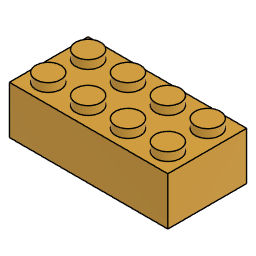
LEGO (Autodesk Fusion 360 design; units mm, degrees)
Autodesk Fusion 360 part; units mm, degrees
sketch "Sketch1" plane through (0, 0, 0) normal (0, 0, 1) x (1, 0, 0) in component "LEGO"
  line L0 (0, 0) -> (31.8, 0)
  line L1 (31.8, 0) -> (31.8, 15.8)
  line L2 (31.8, 15.8) -> (0, 15.8)
  line L3 (0, 15.8) -> (0, 0)
  dimension "d1" = 31.8
  dimension "d2" = 15.8
  constraint horizontal L0
  constraint vertical L1
  constraint horizontal L2
  constraint vertical L3
  constraint coincident L0.start L3.end
  measures "d1" distance of L0.start L0.end
  measures "d2" distance of L0.start L2.end
extrude "Extrude1" add sketch "Sketch1" along normal blind 9.6 makes body 1 in component "LEGO"
sketch "Sketch2" plane through (0, 0, 9.6) normal (0, 0, 1) x (-1, 0, 0) in component "LEGO"
  line L0 (0, -15.8) -> (0, 0)
  line L1 (0, 0) -> (-31.8, 0)
  line L2 (-31.8, 0) -> (-31.8, -15.8)
  line L3 (-31.8, -15.8) -> (0, -15.8)
  circle A0 centre (-3.9, -11.9) radius 2.5
  dimension "d6" = 5
  dimension "d8" = 3.9
  dimension "d10" = 3.9
  measures "d6" diameter of A0
  measures "d8" distance of L3 A0.centre
  measures "d10" distance of L0 A0.centre
extrude "Extrude2" add sketch "Sketch2" along normal blind 1.7 separate body contours A0 makes body 2 in component "LEGO"
pattern_linear "R-Pattern1" count 1 spacing 0 along (0, 0, 1) count 4 spacing 8 along (1, 0, 0) of "Extrude2" makes body 3 makes body 4 makes body 5 in component "LEGO"
pattern_linear "R-Pattern2" count 1 spacing 0 along (1, 0, 0) count 2 spacing 8 along (0, -1, 0) of bodies 2 3 4 5 makes body 6 at (1.4124, 4.1489, 10.1667) makes body 7 at (9.4124, 4.1489, 10.1667) makes body 8 at (17.4124, 4.1489, 10.1667) makes body 9 at (25.4124, 4.1489, 10.1667) in component "LEGO"
shell "Shell1" thickness 1.5 removed faces 1 at (21.2, 5.2667, 0) on bodies 1 in component "LEGO"
component "LEGO" placed x (1, 0, 0) y (0, 1, 0) z (0, 0, 1) at (0, 0, 0)
